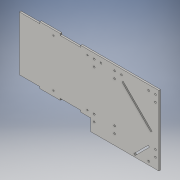
# Autodesk Inventor part: vrRig_v01r1_side
Saved by Autodesk Inventor 2016 (Build 200138000, 138)
## iProperties
Created: 2018-01-13
Part Number: vrRig_v01r1_side
Material: Generic
Document SubType Name: Modeling
Designer: harveylab
Density: 1 g/cm^3
Appearance: Default
Author: harveylab
Autodesk Inventor part; units mm, degrees
ref_plane "YZ Plane" through (0, 0, 0) normal (1, 0, 0) x (0, 1, 0)
ref_plane "XZ Plane" through (0, 0, 0) normal (0, 1, 0) x (-1, 0, 0)
ref_plane "XY Plane" through (0, 0, 0) normal (0, 0, 1) x (1, 0, 0)
sketch "Sketch1" plane through (0, 0, 0) normal (0, 0, 1) x (1, 0, 0)
  circle A0 centre (482.6, 12.7) radius 3.302
  circle A1 centre (508, 241.3) radius 3.302
  circle A2 centre (482.6, 241.3) radius 3.302
  circle A3 centre (355.6, 241.3) radius 3.302
  circle A4 centre (330.2, 241.3) radius 3.302 construction
  circle A5 centre (127, 63.5) radius 3.175 construction
  circle A6 centre (127, 241.3) radius 3.175 construction
  line L0 (427.3692, 9.8745) -> (431.8594, 5.3844)
  line L1 (431.8594, 5.3844) -> (485.7409, 59.2659)
  line L2 (485.7409, 59.2659) -> (481.2508, 63.7561)
  circle A7 centre (330.2, 63.5) radius 3.302 construction
  circle A8 centre (254, 241.3) radius 3.302 construction
  circle A9 centre (279.4, 63.5) radius 3.302
  circle A10 centre (355.6, 63.5) radius 3.302
  circle A11 centre (508, 63.5) radius 3.302
  circle A12 centre (355.6, 12.7) radius 3.302 construction
  circle A13 centre (508, 12.7) radius 3.302 construction
  line L3 (0, 254) -> (76.2, 254)
  line L4 (76.2, 254) -> (76.2, 260.35)
  line L5 (76.2, 260.35) -> (152.4, 260.35)
  line L6 (152.4, 260.35) -> (152.4, 254)
  line L7 (152.4, 254) -> (228.6, 254)
  line L8 (228.6, 254) -> (228.6, 260.35)
  line L9 (228.6, 260.35) -> (520.7, 260.35)
  line L10 (520.7, 260.35) -> (520.7, 0)
  line L11 (520.7, 0) -> (342.9, 0)
  line L12 (228.6, 44.45) -> (228.6, 50.8)
  line L13 (228.6, 50.8) -> (152.4, 50.8)
  line L14 (152.4, 50.8) -> (152.4, 44.45)
  line L15 (152.4, 44.45) -> (76.2, 44.45)
  line L16 (76.2, 44.45) -> (76.2, 50.8)
  line L17 (76.2, 50.8) -> (0, 50.8)
  line L18 (0, 50.8) -> (0, 254)
  line L19 (490.8349, 111.3178) -> (383.0718, 219.0809)
  line L20 (383.0718, 219.0809) -> (387.562, 223.571)
  line L21 (387.562, 223.571) -> (495.3, 115.7829)
  line L22 (495.3, 115.7829) -> (490.8349, 111.3178)
  line L23 (427.3692, 9.8745) -> (481.2508, 63.7561)
  circle A14 centre (279.4, 241.3) radius 3.302
  circle A15 centre (381, 241.3) radius 3.302
  circle A16 centre (254, 63.5) radius 3.302 construction
  circle A17 centre (304.8, 241.3) radius 3.302
  circle A18 centre (304.8, 63.5) radius 3.302 construction
  line L24 (266.7, 0) -> (342.9, 0)
  line L25 (266.7, 0) -> (266.7, 44.45)
  line L26 (228.6, 44.45) -> (266.7, 44.45)
  circle A19 centre (279.4, 12.7) radius 3.302 construction
  line L27 (279.4, 12.7) -> (279.4, 38.1) construction
  line L28 (279.4, 38.1) -> (304.8, 38.1) construction
  line L29 (304.8, 38.1) -> (355.6, 38.1) construction
  circle A20 centre (355.6, 38.1) radius 3.302
  circle A21 centre (279.4, 38.1) radius 3.302
  line L30 (508, 12.7) -> (508, 38.1) construction
  circle A22 centre (508, 38.1) radius 3.302
  line L31 (508, 241.3) -> (508, 215.9) construction
  line L32 (355.6, 241.3) -> (355.6, 215.9) construction
  line L33 (279.4, 241.3) -> (279.4, 215.9) construction
  circle A23 centre (279.4, 215.9) radius 3.302
  circle A24 centre (355.6, 215.9) radius 3.302
  circle A25 centre (508, 215.9) radius 3.302
  point P0 (0, 0)
  dimension "d6" = 25.4
  dimension "d7" = 25.4
  constraints: 68 end point, 26 centre point, 5 vertical, 1 coincident, 1 horizontal, 1 perpendicular, 1 point on line
  measures "d6" distance of L27.start L27.end
  measures "d7" distance of L31.start L31.end
sketch "Sketch2" plane through (0, 0, 0) normal (0, 0, 1) x (1, 0, 0)
  point P0 (0, 0)
  point P1 (127, 241.3)
  point P2 (127, 63.5)
  point P3 (254, 63.5)
  point P4 (254, 241.3)
extrude "Extrusion4" add sketch "Sketch1" along normal blind 6.35
hole "Hole2" at (127, 241.3, 0) at (127, 63.5, 0) at (254, 63.5, 0) at (254, 241.3, 0) direction (0, 0, 1) diameter 4.9784 depth 19.05 tip angle 118 thread size "1/4-20 UNC" class "2B" standard "ANSI Unified Screw Threads"
body "Solid3"
